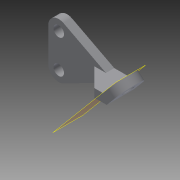
# Autodesk Inventor part: 零件7-20
Saved by Autodesk Inventor 2014 (Build 180170000, 170)
## iProperties
Created: 2018-12-21
Part Number: 零件7-20
Material: 常规
Document SubType Name: Modeling
Designer: Administrator
Density: 1 g/cm^3
Appearance: 默认
Author: Administrator
Autodesk Inventor part; units mm, degrees
ref_plane "YZ Plane" through (0, 0, 0) normal (1, 0, 0) x (0, 1, 0)
ref_plane "XZ Plane" through (0, 0, 0) normal (0, 1, 0) x (-1, 0, 0)
sketch "草图1" plane through (0, 0, 0) normal (0, 1, 0) x (-1, 0, 0)
  line L0 (55.5004, 0) -> (-70.183, 0)
  line L1 (21.9957, -8) -> (21.9957, 8)
  line L2 (14.6949, 12.4392) -> (-9.3051, 0)
  line L3 (14.6949, -12.4392) -> (-9.3051, 0)
  arc A0 (14.6949, -12.4392) -> (21.9957, -8) centre (16.9957, -8) ccw
  arc A1 (21.9957, 8) -> (14.6949, 12.4392) centre (16.9957, 8) ccw
  circle A2 centre (16.9957, -8) radius 2.5
  circle A3 centre (16.9957, 8) radius 2.5
  point P0 (0, 0)
  dimension "d0" = 5
  dimension "d1" = 16
  dimension "d2" = 24
  dimension "d3" = 5
  dimension "d4" = 5
  constraints: 8 end point, 4 centre point, 4 point on circle, 4 tangent, 2 coincident, 2 point on line, 1 equal radius, 1 horizontal, 1 perpendicular, 1 other
  measures "d0" radius of A0
  measures "d1" distance of L1.start L1.end
  measures "d2" horizontal distance of L2.start L2.end
  measures "d3" diameter of A2
  measures "d4" diameter of A3
extrude "拉伸1" add sketch "草图1" along normal blind 4
sketch "草图2" plane through (0, 0, 0) normal (0, 0, 1) x (1, 0, 0)
  line L0 (9.3051, 0) -> (-14.6949, 0) projected
  line L1 (9.3051, 0) -> (9.3051, 4) projected
  line L2 (-14.6949, 4) -> (9.3051, 4) projected
  line L3 (-14.6949, 0) -> (-14.6949, 4) projected
  line L4 (0, 4) -> (13, 4)
  line L5 (13, 4) -> (13, -9)
  line L6 (13, -9) -> (9, -9)
  line L7 (9, -9) -> (0, 0)
  line L8 (0, 0) -> (0, 4)
  dimension "d7" = 13
  dimension "d8" = 13
  dimension "d9" = 4
  constraints: 10 end point, 3 perpendicular, 2 point on line
  measures "d7" distance of L4.start L4.end
  measures "d8" distance of L4.end L5.end
  measures "d9" distance of L5.end L6.end
extrude "拉伸2" add sketch "草图2" along normal mid plane 4 contours L1 L4 L5 L6 L7 L0 | L0 L8 L2 L1
ref_plane "工作平面1" through (13, -9, 2) normal (0.7660444, 0, -0.6427876) x (0, 1, 0)
sketch "草图3" plane through (13, -9, 2) normal (0.7660444, 0, -0.6427876) x (0, 1, 0)
  line L0 (13, -3.0642) -> (13, 0) projected
  line L1 (0, 0) -> (13, 0) projected
  line L2 (0, -3.0642) -> (0, 0) projected
  line L3 (13, -3.0642) -> (0, -3.0642) projected
  line L4 (9, -7.9196) -> (9, -11.4204) projected
  line L5 (13, -7.9196) -> (9, -7.9196) projected
  line L6 (13, -7.9196) -> (13, -3.0642) projected
  line L7 (13, -3.0642) -> (0, -3.0642) projected
  line L8 (0, -3.0642) -> (0, -5.6353) projected
  line L9 (0, -5.6353) -> (9, -11.4204) projected
  line L10 (0, -3.0642) -> (13, -3.0642)
  line L11 (13, -3.0642) -> (13, 3.9358)
  line L12 (0, 3.9358) -> (0, -3.0642)
  arc A0 (13, 3.9358) -> (0, 3.9358) centre (6.5, 3.9358) ccw
  circle A1 centre (6.5, 3.9358) radius 2.5
  point P0 (9, -9.8883)
  dimension "d13" = 6.5
  dimension "d14" = 7
  dimension "d15" = 5
  constraints: 6 end point, 2 centre point, 2 point on circle, 2 tangent, 1 coincident, 1 horizontal, 1 parallel, 1 perpendicular
  measures "d13" radius of A0
  measures "d14" distance of L12.start L7.end
  measures "d15" diameter of A1
extrude "拉伸3" add sketch "草图3" along normal blind 4 contours L3 L2 L1 L0 | L1 L12 A0 L11
sketch "草图4" plane through (0, 4, 0) normal (0, 1, 0) x (1, 0, 0)
  line L0 (13, -2) -> (5.4463, -2) projected
  line L1 (14.0946, 2.9184) -> (18.5941, -2.4439) projected
  line L2 (13, 2) -> (14.0946, 2.9184) projected
  line L3 (13, 2) -> (14.8652, 2)
  point P0 (0, 0)
  constraints: 2 end point, 1 parallel, 1 point on line
extrude "拉伸4" cut sketch "草图4" against normal blind 20
